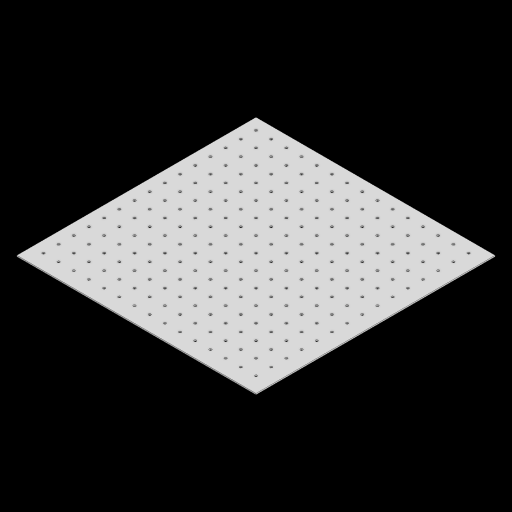
# Autodesk Inventor part: mounting_board
Saved by Autodesk Inventor 2023 (Build 270158000, 158)
## iProperties
Created: 2024-07-03
Part Number: mounting_board
Material: 일반
Document SubType Name: Modeling
Designer: OMS55
Density: 1 g/cm^3
Appearance: 기본값
Author: OMS55
Autodesk Inventor part; units mm, degrees
ref_plane "YZ Plane" through (0, 0, 0) normal (1, 0, 0) x (0, 1, 0)
ref_plane "XZ Plane" through (0, 0, 0) normal (0, 1, 0) x (-1, 0, 0)
ref_plane "XY Plane" through (0, 0, 0) normal (0, 0, 1) x (1, 0, 0)
sketch "스케치1" plane through (0, 0, 0) normal (0, 1, 0) x (-1, 0, 0)
  line L0 (0, 0) -> (400, 0)
  line L1 (400, 0) -> (400, -400)
  line L2 (400, -400) -> (0, -400)
  line L3 (0, -400) -> (0, 0)
  circle A0 centre (25.4, -25.4) radius 2.0475
  circle A1 centre (25.4, -50.8) radius 2.0475
  circle A2 centre (25.4, -76.2) radius 2.0475
  circle A3 centre (25.4, -101.6) radius 2.0475
  circle A4 centre (25.4, -127) radius 2.0475
  circle A5 centre (25.4, -152.4) radius 2.0475
  circle A6 centre (25.4, -177.8) radius 2.0475
  circle A7 centre (25.4, -203.2) radius 2.0475
  circle A8 centre (25.4, -228.6) radius 2.0475
  circle A9 centre (25.4, -254) radius 2.0475
  circle A10 centre (25.4, -279.4) radius 2.0475
  circle A11 centre (25.4, -304.8) radius 2.0475
  circle A12 centre (25.4, -330.2) radius 2.0475
  circle A13 centre (25.4, -355.6) radius 2.0475
  circle A14 centre (25.4, -381) radius 2.0475
  circle A15 centre (50.8, -25.4) radius 2.0475
  circle A16 centre (50.8, -50.8) radius 2.0475
  circle A17 centre (50.8, -76.2) radius 2.0475
  circle A18 centre (50.8, -101.6) radius 2.0475
  circle A19 centre (50.8, -127) radius 2.0475
  circle A20 centre (50.8, -152.4) radius 2.0475
  circle A21 centre (50.8, -177.8) radius 2.0475
  circle A22 centre (50.8, -203.2) radius 2.0475
  circle A23 centre (50.8, -228.6) radius 2.0475
  circle A24 centre (50.8, -254) radius 2.0475
  circle A25 centre (50.8, -279.4) radius 2.0475
  circle A26 centre (50.8, -304.8) radius 2.0475
  circle A27 centre (50.8, -330.2) radius 2.0475
  circle A28 centre (50.8, -355.6) radius 2.0475
  circle A29 centre (50.8, -381) radius 2.0475
  circle A30 centre (76.2, -25.4) radius 2.0475
  circle A31 centre (76.2, -50.8) radius 2.0475
  circle A32 centre (76.2, -76.2) radius 2.0475
  circle A33 centre (76.2, -101.6) radius 2.0475
  circle A34 centre (76.2, -127) radius 2.0475
  circle A35 centre (76.2, -152.4) radius 2.0475
  circle A36 centre (76.2, -177.8) radius 2.0475
  circle A37 centre (76.2, -203.2) radius 2.0475
  circle A38 centre (76.2, -228.6) radius 2.0475
  circle A39 centre (76.2, -254) radius 2.0475
  circle A40 centre (76.2, -279.4) radius 2.0475
  circle A41 centre (76.2, -304.8) radius 2.0475
  circle A42 centre (76.2, -330.2) radius 2.0475
  circle A43 centre (76.2, -355.6) radius 2.0475
  circle A44 centre (76.2, -381) radius 2.0475
  circle A45 centre (101.6, -25.4) radius 2.0475
  circle A46 centre (101.6, -50.8) radius 2.0475
  circle A47 centre (101.6, -76.2) radius 2.0475
  circle A48 centre (101.6, -101.6) radius 2.0475
  circle A49 centre (101.6, -127) radius 2.0475
  circle A50 centre (101.6, -152.4) radius 2.0475
  circle A51 centre (101.6, -177.8) radius 2.0475
  circle A52 centre (101.6, -203.2) radius 2.0475
  circle A53 centre (101.6, -228.6) radius 2.0475
  circle A54 centre (101.6, -254) radius 2.0475
  circle A55 centre (101.6, -279.4) radius 2.0475
  circle A56 centre (101.6, -304.8) radius 2.0475
  circle A57 centre (101.6, -330.2) radius 2.0475
  circle A58 centre (101.6, -355.6) radius 2.0475
  circle A59 centre (101.6, -381) radius 2.0475
  circle A60 centre (127, -25.4) radius 2.0475
  circle A61 centre (127, -50.8) radius 2.0475
  circle A62 centre (127, -76.2) radius 2.0475
  circle A63 centre (127, -101.6) radius 2.0475
  circle A64 centre (127, -127) radius 2.0475
  circle A65 centre (127, -152.4) radius 2.0475
  circle A66 centre (127, -177.8) radius 2.0475
  circle A67 centre (127, -203.2) radius 2.0475
  circle A68 centre (127, -228.6) radius 2.0475
  circle A69 centre (127, -254) radius 2.0475
  circle A70 centre (127, -279.4) radius 2.0475
  circle A71 centre (127, -304.8) radius 2.0475
  circle A72 centre (127, -330.2) radius 2.0475
  circle A73 centre (127, -355.6) radius 2.0475
  circle A74 centre (127, -381) radius 2.0475
  circle A75 centre (152.4, -25.4) radius 2.0475
  circle A76 centre (152.4, -50.8) radius 2.0475
  circle A77 centre (152.4, -76.2) radius 2.0475
  circle A78 centre (152.4, -101.6) radius 2.0475
  circle A79 centre (152.4, -127) radius 2.0475
  circle A80 centre (152.4, -152.4) radius 2.0475
  circle A81 centre (152.4, -177.8) radius 2.0475
  circle A82 centre (152.4, -203.2) radius 2.0475
  circle A83 centre (152.4, -228.6) radius 2.0475
  circle A84 centre (152.4, -254) radius 2.0475
  circle A85 centre (152.4, -279.4) radius 2.0475
  circle A86 centre (152.4, -304.8) radius 2.0475
  circle A87 centre (152.4, -330.2) radius 2.0475
  circle A88 centre (152.4, -355.6) radius 2.0475
  circle A89 centre (152.4, -381) radius 2.0475
  circle A90 centre (177.8, -25.4) radius 2.0475
  circle A91 centre (177.8, -50.8) radius 2.0475
  circle A92 centre (177.8, -76.2) radius 2.0475
  circle A93 centre (177.8, -101.6) radius 2.0475
  circle A94 centre (177.8, -127) radius 2.0475
  circle A95 centre (177.8, -152.4) radius 2.0475
  circle A96 centre (177.8, -177.8) radius 2.0475
  circle A97 centre (177.8, -203.2) radius 2.0475
  circle A98 centre (177.8, -228.6) radius 2.0475
  circle A99 centre (177.8, -254) radius 2.0475
  circle A100 centre (177.8, -279.4) radius 2.0475
  circle A101 centre (177.8, -304.8) radius 2.0475
  circle A102 centre (177.8, -330.2) radius 2.0475
  circle A103 centre (177.8, -355.6) radius 2.0475
  circle A104 centre (177.8, -381) radius 2.0475
  circle A105 centre (203.2, -25.4) radius 2.0475
  circle A106 centre (203.2, -50.8) radius 2.0475
  circle A107 centre (203.2, -76.2) radius 2.0475
  circle A108 centre (203.2, -101.6) radius 2.0475
  circle A109 centre (203.2, -127) radius 2.0475
  circle A110 centre (203.2, -152.4) radius 2.0475
  circle A111 centre (203.2, -177.8) radius 2.0475
  circle A112 centre (203.2, -203.2) radius 2.0475
  circle A113 centre (203.2, -228.6) radius 2.0475
  circle A114 centre (203.2, -254) radius 2.0475
  circle A115 centre (203.2, -279.4) radius 2.0475
  circle A116 centre (203.2, -304.8) radius 2.0475
  circle A117 centre (203.2, -330.2) radius 2.0475
  circle A118 centre (203.2, -355.6) radius 2.0475
  circle A119 centre (203.2, -381) radius 2.0475
  circle A120 centre (228.6, -25.4) radius 2.0475
  circle A121 centre (228.6, -50.8) radius 2.0475
  circle A122 centre (228.6, -76.2) radius 2.0475
  circle A123 centre (228.6, -101.6) radius 2.0475
  circle A124 centre (228.6, -127) radius 2.0475
  circle A125 centre (228.6, -152.4) radius 2.0475
  circle A126 centre (228.6, -177.8) radius 2.0475
  circle A127 centre (228.6, -203.2) radius 2.0475
  circle A128 centre (228.6, -228.6) radius 2.0475
  circle A129 centre (228.6, -254) radius 2.0475
  circle A130 centre (228.6, -279.4) radius 2.0475
  circle A131 centre (228.6, -304.8) radius 2.0475
  circle A132 centre (228.6, -330.2) radius 2.0475
  circle A133 centre (228.6, -355.6) radius 2.0475
  circle A134 centre (228.6, -381) radius 2.0475
  circle A135 centre (254, -25.4) radius 2.0475
  circle A136 centre (254, -50.8) radius 2.0475
  circle A137 centre (254, -76.2) radius 2.0475
  circle A138 centre (254, -101.6) radius 2.0475
  circle A139 centre (254, -127) radius 2.0475
  circle A140 centre (254, -152.4) radius 2.0475
  circle A141 centre (254, -177.8) radius 2.0475
  circle A142 centre (254, -203.2) radius 2.0475
  circle A143 centre (254, -228.6) radius 2.0475
  circle A144 centre (254, -254) radius 2.0475
  circle A145 centre (254, -279.4) radius 2.0475
  circle A146 centre (254, -304.8) radius 2.0475
  circle A147 centre (254, -330.2) radius 2.0475
  circle A148 centre (254, -355.6) radius 2.0475
  circle A149 centre (254, -381) radius 2.0475
  circle A150 centre (279.4, -25.4) radius 2.0475
  circle A151 centre (279.4, -50.8) radius 2.0475
  circle A152 centre (279.4, -76.2) radius 2.0475
  circle A153 centre (279.4, -101.6) radius 2.0475
  circle A154 centre (279.4, -127) radius 2.0475
  circle A155 centre (279.4, -152.4) radius 2.0475
  circle A156 centre (279.4, -177.8) radius 2.0475
  circle A157 centre (279.4, -203.2) radius 2.0475
  circle A158 centre (279.4, -228.6) radius 2.0475
  circle A159 centre (279.4, -254) radius 2.0475
  circle A160 centre (279.4, -279.4) radius 2.0475
  circle A161 centre (279.4, -304.8) radius 2.0475
  circle A162 centre (279.4, -330.2) radius 2.0475
  circle A163 centre (279.4, -355.6) radius 2.0475
  circle A164 centre (279.4, -381) radius 2.0475
  circle A165 centre (304.8, -25.4) radius 2.0475
  circle A166 centre (304.8, -50.8) radius 2.0475
  circle A167 centre (304.8, -76.2) radius 2.0475
  circle A168 centre (304.8, -101.6) radius 2.0475
  circle A169 centre (304.8, -127) radius 2.0475
  circle A170 centre (304.8, -152.4) radius 2.0475
  circle A171 centre (304.8, -177.8) radius 2.0475
  circle A172 centre (304.8, -203.2) radius 2.0475
  circle A173 centre (304.8, -228.6) radius 2.0475
  circle A174 centre (304.8, -254) radius 2.0475
  circle A175 centre (304.8, -279.4) radius 2.0475
  circle A176 centre (304.8, -304.8) radius 2.0475
  circle A177 centre (304.8, -330.2) radius 2.0475
  circle A178 centre (304.8, -355.6) radius 2.0475
  circle A179 centre (304.8, -381) radius 2.0475
  circle A180 centre (330.2, -25.4) radius 2.0475
  circle A181 centre (330.2, -50.8) radius 2.0475
  circle A182 centre (330.2, -76.2) radius 2.0475
  circle A183 centre (330.2, -101.6) radius 2.0475
  circle A184 centre (330.2, -127) radius 2.0475
  circle A185 centre (330.2, -152.4) radius 2.0475
  circle A186 centre (330.2, -177.8) radius 2.0475
  circle A187 centre (330.2, -203.2) radius 2.0475
  circle A188 centre (330.2, -228.6) radius 2.0475
  circle A189 centre (330.2, -254) radius 2.0475
  circle A190 centre (330.2, -279.4) radius 2.0475
  circle A191 centre (330.2, -304.8) radius 2.0475
  circle A192 centre (330.2, -330.2) radius 2.0475
  circle A193 centre (330.2, -355.6) radius 2.0475
  circle A194 centre (330.2, -381) radius 2.0475
  circle A195 centre (355.6, -25.4) radius 2.0475
  circle A196 centre (355.6, -50.8) radius 2.0475
  circle A197 centre (355.6, -76.2) radius 2.0475
  circle A198 centre (355.6, -101.6) radius 2.0475
  circle A199 centre (355.6, -127) radius 2.0475
  circle A200 centre (355.6, -152.4) radius 2.0475
  circle A201 centre (355.6, -177.8) radius 2.0475
  circle A202 centre (355.6, -203.2) radius 2.0475
  circle A203 centre (355.6, -228.6) radius 2.0475
  circle A204 centre (355.6, -254) radius 2.0475
  circle A205 centre (355.6, -279.4) radius 2.0475
  circle A206 centre (355.6, -304.8) radius 2.0475
  circle A207 centre (355.6, -330.2) radius 2.0475
  circle A208 centre (355.6, -355.6) radius 2.0475
  circle A209 centre (355.6, -381) radius 2.0475
  circle A210 centre (381, -25.4) radius 2.0475
  circle A211 centre (381, -50.8) radius 2.0475
  circle A212 centre (381, -76.2) radius 2.0475
  circle A213 centre (381, -101.6) radius 2.0475
  circle A214 centre (381, -127) radius 2.0475
  circle A215 centre (381, -152.4) radius 2.0475
  circle A216 centre (381, -177.8) radius 2.0475
  circle A217 centre (381, -203.2) radius 2.0475
  circle A218 centre (381, -228.6) radius 2.0475
  circle A219 centre (381, -254) radius 2.0475
  circle A220 centre (381, -279.4) radius 2.0475
  circle A221 centre (381, -304.8) radius 2.0475
  circle A222 centre (381, -330.2) radius 2.0475
  circle A223 centre (381, -355.6) radius 2.0475
  circle A224 centre (381, -381) radius 2.0475
  dimension "d0" = 400
  dimension "d1" = 400
  dimension "d2" = 25.4
  dimension "d3" = 25.4
  dimension "d4" = 4.095
  dimension "d7" = 25.4
  dimension "d10" = 25.4
  constraints: 225 centre point, 8 end point, 2 horizontal, 2 parallel, 1 coincident, 1 perpendicular, 1 vertical, 448 other
  measures "d0" distance of L2.end L0.start
  measures "d1" distance of L1.end L2.end
  measures "d2" distance from line of L3 A0.centre
  measures "d3" distance from line of L0 A0.centre
  measures "d4" diameter of A0
  measures "d7" distance of A0.centre A1.centre
  measures "d10" distance of A0.centre A15.centre
extrude "돌출1" add sketch "스케치1" along normal blind 2
